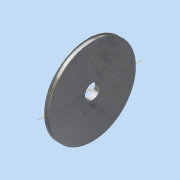
# Autodesk Inventor part: Rad d72 b4 r3.5
Saved by Autodesk Inventor 2015 (Build 190159000, 159)
## iProperties
Created: 2017-11-10
Part Number: Rad d72 b4 r3.5
Material: Generisch
Document SubType Name: Modeling
Designer: Christoph Soppa
Density: 1 g/cm^3
Appearance: Aluminium - poliert
Author: Christoph Soppa
Autodesk Inventor part; units mm, degrees
ref_plane "YZ Plane" through (0, 0, 0) normal (1, 0, 0) x (0, 1, 0)
ref_plane "XZ Plane" through (0, 0, 0) normal (0, 1, 0) x (-1, 0, 0)
ref_plane "XY Plane" through (0, 0, 0) normal (0, 0, 1) x (1, 0, 0)
sketch "Skizze2" plane through (0, 0, 0) normal (0, 0, 1) x (1, 0, 0)
  line L0 (-2, 6) -> (2, 6)
  line L1 (2, 6) -> (2, 35.25)
  line L2 (2, 35.25) -> (1.75, 35.25)
  line L3 (-2, 6) -> (-2, 35.25)
  line L4 (-2, 35.25) -> (-1.75, 35.25)
  arc A0 (-1.75, 35.25) -> (1.75, 35.25) centre (0, 35.25) ccw
  line L5 (-5.378, 0) -> (18.2681, 0) projected
  line L6 (0, -7.05) -> (0, 42.3) projected
  line L7 (-1.44, 0) -> (14.8901, 0)
  point P0 (0, 0)
  dimension "d2" = 1.75
  dimension "d3" = 6
  dimension "d4" = 2
  dimension "d5" = 4
  dimension "d6" = 0.25
  dimension "d7" = 0.25
  dimension "d12" = 29.25
  dimension "d13" = 29.25
  dimension "d14" = 14.8901
  dimension "d15" = 1.44
  constraints: 12 end point, 3 perpendicular, 2 point on circle, 2 point on line, 1 centre point, 1 horizontal, 1 vertical
  measures "d2" radius of A0
  measures "d3" distance from line of point (0, 0) L0
  measures "d4" distance from line of point (0, 0) L3
  measures "d5" distance of L0.start L0.end
  measures "d6" distance of L3.end L4.end
  measures "d7" distance of L1.end L2.end
  measures "d12" distance of L0.end L1.end
  measures "d13" distance of L0.start L3.end
  measures "d14" distance from line of L7.end L6
  measures "d15" distance from line of L7.start L6
revolve "Umdrehung1" add sketch "Skizze2" angle 360 about axis through (-1.44, 0, 0) along (1, 0, 0)
